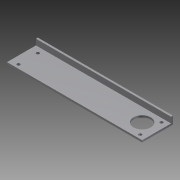
# Autodesk Inventor part: 8 ball bottom 1 by 2 L short
Saved by Autodesk Inventor 2012 (Build 160160000, 160)
## iProperties
Created: 2013-10-10
Part Number: 8 ball bottom 1 by 2 L short
Material: Default
Document SubType Name: Modeling
Designer: Bryce
Density: 1 g/cm^3
Author: Bryce
Autodesk Inventor part; units mm, degrees
ref_plane "YZ Plane" through (0, 0, 0) normal (1, 0, 0) x (0, 1, 0)
ref_plane "XZ Plane" through (0, 0, 0) normal (0, 1, 0) x (-1, 0, 0)
ref_plane "XY Plane" through (0, 0, 0) normal (0, 0, 1) x (1, 0, 0)
sketch "Sketch1" plane through (0, 0, 0) normal (0, 0, 1) x (1, 0, 0)
  line L0 (0, 0) -> (222.25, 0)
  line L1 (0, 0) -> (0, 3.175)
  line L2 (0, 3.175) -> (222.25, 3.175)
  line L3 (0, 3.175) -> (0, 12.7)
  line L4 (0, 12.7) -> (222.25, 12.7)
  line L5 (222.25, 0) -> (222.25, 12.7)
  dimension "d4" = 3.175
  dimension "d9" = 12.7
  dimension "d11" = 222.25
  constraints: 12 end point, 5 perpendicular, 1 horizontal, 1 point on line
  measures "d4" distance of L0.start L1.end
  measures "d9" distance between parallel lines of L4 L0
  measures "d11" distance of L0.start L0.end
extrude "Extrusion1" add sketch "Sketch1" along normal blind 3.175
extrude "Extrusion2" add sketch "Sketch1" along normal blind 50.8 contours L1 L2 L5 L0
sketch "Sketch2" plane through (0, 0, 0) normal (0, -1, 0) x (1, 0, 0)
  circle A0 centre (196.85, 25.4) radius 14.2875
  line L0 (0, 0) -> (0, 50.8) projected
  line L1 (0, 0) -> (222.25, 0) projected
  line L2 (222.25, 0) -> (222.25, 50.8) projected
  line L3 (222.25, 50.8) -> (0, 50.8) projected
  circle A1 centre (12.7, 44.45) radius 2.54
  circle A2 centre (12.7, 12.7) radius 2.54
  circle A3 centre (212.725, 44.45) radius 2.54
  circle A4 centre (212.725, 9.525) radius 2.54
  dimension "d26" = 25.4
  dimension "d27" = 25.4
  dimension "d28" = 28.575
  dimension "d29" = 5.08
  dimension "d30" = 12.7
  dimension "d31" = 6.35
  dimension "d32" = 12.7
  dimension "d33" = 12.7
  dimension "d34" = 6.35
  dimension "d35" = 9.525
  dimension "d36" = 9.525
  dimension "d37" = 9.525
  constraints: 5 centre point, 3 equal radius
  measures "d26" distance from line of L2 A0.centre
  measures "d27" distance from line of L3 A0.centre
  measures "d28" diameter of A0
  measures "d29" diameter of A1
  measures "d30" distance from line of L0 A2.centre
  measures "d31" distance from line of L3 A1.centre
  measures "d32" distance from line of L0 A1.centre
  measures "d33" distance from line of L1 A2.centre
  measures "d34" distance from line of L3 A3.centre
  measures "d35" distance from line of L2 A3.centre
  measures "d36" distance from line of A4.centre L2
  measures "d37" distance from line of L1 A4.centre
extrude "Extrusion3" cut sketch "Sketch2" against normal through all contours A0 | A1 | A2 | A3 | A4
equation "\"d4\" = d6"
equation "\"d30\" = d32"
equation "\"d34\" = d31"
equation "\"d36\" = d35"
equation "\"d6\" = 3.175"
body "Solid1"
